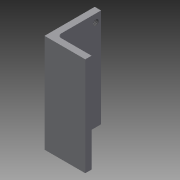
# Autodesk Inventor part: Left Angle
Saved by Autodesk Inventor 2013 (Build 170138000, 138)
## iProperties
Created: 2012-09-25
Part Number: Left Angle
Material: Generic
Document SubType Name: Modeling
Designer: uqgtayle
Density: 1 g/cm^3
Author: uqgtayle
Autodesk Inventor part; units mm, degrees
ref_plane "YZ Plane" through (0, 0, 0) normal (1, 0, 0) x (0, 1, 0)
ref_plane "XZ Plane" through (0, 0, 0) normal (0, 1, 0) x (-1, 0, 0)
ref_plane "XY Plane" through (0, 0, 0) normal (0, 0, 1) x (1, 0, 0)
sketch "Sketch1" plane through (0, 0, 0) normal (0, 0, 1) x (1, 0, 0)
  line L0 (0, 38.2) -> (0, 0)
  line L1 (0, 0) -> (31, 0)
  line L2 (31, 0) -> (31, 4.8)
  line L3 (31, 4.8) -> (7.8, 4.8)
  line L4 (4.8, 7.8) -> (4.8, 38.2)
  line L5 (4.8, 38.2) -> (0, 38.2)
  arc A0 (4.8, 7.8) -> (7.8, 4.8) centre (7.8, 7.8) ccw
  dimension "d0" = 31
  dimension "d1" = 38.2
  dimension "d2" = 4.8
  dimension "d3" = 4.8
  dimension "d4" = 3
  constraints: 12 end point, 4 parallel, 2 point on circle, 2 tangent, 1 centre point, 1 perpendicular, 1 vertical
  measures "d0" distance of L1.end L0.end
  measures "d1" distance of L0.start L0.end
  measures "d2" distance of L1.end L2.end
  measures "d3" distance of L0.start L4.end
  measures "d4" radius of A0
extrude "Extrusion1" add sketch "Sketch1" against normal blind 75
sketch "Sketch2" plane through (0, 0, 0) normal (-1, 0, 0) x (0, 0, 1)
  line L0 (0, 0) -> (0, 38.2) projected
  line L1 (0, 38.2) -> (-75, 38.2) projected
  point P0 (-6, 34.2)
  dimension "d7" = 4
  dimension "d8" = 6
  measures "d7" distance from line of L1 point (-6, 34.2)
  measures "d8" distance from line of point (-6, 34.2) L0
hole "Hole1" at (0, 34.2, -6) direction (1, 0, 0) diameter 4.134 end through all thread size "M5x0.8" class "6H" standard "ANSI Metric M Profile"
body "Solid1"
